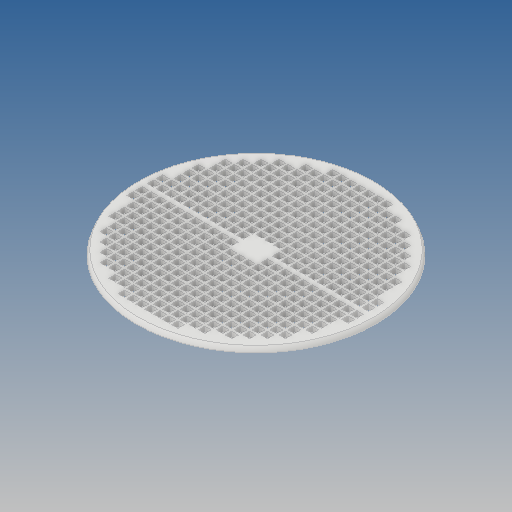
# Autodesk Inventor part: тело
Saved by Autodesk Inventor 2020 (Build 240168000, 168)
## iProperties
Created: 2019-09-06
Part Number: тело
Material: Пластик АБС
Document SubType Name: Modeling
Designer: Iliga
Density: 1.06 g/cm^3
Appearance: Гладкий — белый
Mass: 236.83 g
Surface Area: 2382.33 cm^2
Volume: 236.83 cm^3
Author: Iliga
Autodesk Inventor part; units mm, degrees
(part 1 of 3)
ref_plane "РабПлоскость1" through (0, -35, 0) normal (0, 1, 0) x (-1, 0, 0)
ref_plane "РабПлоскость7" through (100, -35, 0) normal (0, -1, 0) x (1, 0, 0)
ref_plane "YZ Plane" through (0, 0, 0) normal (1, 0, 0) x (0, 1, 0)
sketch "Эскиз118" plane through (0, 0, 0) normal (0, 0, 1) x (1, 0, 0)
  line L0 (0, 0) -> (-93.5, 0)
  line L1 (0, 4) -> (-91.9721, 4)
  line L2 (0, 4) -> (0, 0)
  line L3 (0, 45) -> (0, -57)
  arc A0 (-91.9721, 4) -> (-93.5, 0) centre (-87.5, 0) ccw
  point P0 (0, 2)
  dimension "d610" = 93.5
  dimension "d611" = 4
  dimension "d745" = 6
  constraints: 8 end point, 2 horizontal, 2 point on circle, 2 point on line, 2 vertical, 1 centre point, 1 midpoint
  measures "d610" distance of L0.start L0.end
  measures "d611" distance between parallel lines of L0 L1
  measures "d745" radius of A0
revolve "Вращение3" add sketch "Эскиз118" angle 270 about axis through (0, 45, 0) along (0, -1, 0)
sketch "Эскиз119" plane through (-91.9721, 4, 0) normal (0, 1, 0) x (1, 0, 0)
  line L0 (4.9721, 2) -> (9.9721, 2)
  line L1 (9.9721, 2) -> (9.9721, 7)
  line L2 (9.9721, 7) -> (4.9721, 7)
  line L3 (4.9721, 7) -> (4.9721, 2)
  line L4 (0, 0) -> (91.9721, 0) projected
  line L5 (91.9721, -91.9721) -> (91.9721, 0) projected
  line L6 (11.9721, 2) -> (16.9721, 2)
  line L7 (16.9721, 2) -> (16.9721, 7)
  line L8 (16.9721, 7) -> (11.9721, 7)
  line L9 (11.9721, 7) -> (11.9721, 2)
  line L10 (18.9721, 2) -> (23.9721, 2)
  line L11 (23.9721, 2) -> (23.9721, 7)
  line L12 (23.9721, 7) -> (18.9721, 7)
  line L13 (18.9721, 7) -> (18.9721, 2)
  line L14 (25.9721, 2) -> (30.9721, 2)
  line L15 (30.9721, 2) -> (30.9721, 7)
  line L16 (30.9721, 7) -> (25.9721, 7)
  line L17 (25.9721, 7) -> (25.9721, 2)
  line L18 (32.9721, 2) -> (37.9721, 2)
  line L19 (37.9721, 2) -> (37.9721, 7)
  line L20 (37.9721, 7) -> (32.9721, 7)
  line L21 (32.9721, 7) -> (32.9721, 2)
  line L22 (39.9721, 2) -> (44.9721, 2)
  line L23 (44.9721, 2) -> (44.9721, 7)
  line L24 (44.9721, 7) -> (39.9721, 7)
  line L25 (39.9721, 7) -> (39.9721, 2)
  line L26 (46.9721, 2) -> (51.9721, 2)
  line L27 (51.9721, 2) -> (51.9721, 7)
  line L28 (51.9721, 7) -> (46.9721, 7)
  line L29 (46.9721, 7) -> (46.9721, 2)
  line L30 (53.9721, 2) -> (58.9721, 2)
  line L31 (58.9721, 2) -> (58.9721, 7)
  line L32 (58.9721, 7) -> (53.9721, 7)
  line L33 (53.9721, 7) -> (53.9721, 2)
  line L34 (60.9721, 2) -> (65.9721, 2)
  line L35 (65.9721, 2) -> (65.9721, 7)
  line L36 (65.9721, 7) -> (60.9721, 7)
  line L37 (60.9721, 7) -> (60.9721, 2)
  line L38 (67.9721, 2) -> (72.9721, 2)
  line L39 (72.9721, 2) -> (72.9721, 7)
  line L40 (72.9721, 7) -> (67.9721, 7)
  line L41 (67.9721, 7) -> (67.9721, 2)
  line L42 (74.9721, 2) -> (79.9721, 2)
  line L43 (79.9721, 2) -> (79.9721, 7)
  line L44 (79.9721, 7) -> (74.9721, 7)
  line L45 (74.9721, 7) -> (74.9721, 2)
  line L46 (81.9721, 2) -> (86.9721, 2)
  line L47 (86.9721, 2) -> (86.9721, 7)
  line L48 (86.9721, 7) -> (81.9721, 7)
  line L49 (81.9721, 7) -> (81.9721, 2)
  line L50 (88.9721, 2) -> (93.9721, 2)
  line L51 (93.9721, 2) -> (93.9721, 7)
  line L52 (93.9721, 7) -> (88.9721, 7)
  line L53 (88.9721, 7) -> (88.9721, 2)
  line L54 (95.9721, 2) -> (100.9721, 2)
  line L55 (100.9721, 2) -> (100.9721, 7)
  line L56 (100.9721, 7) -> (95.9721, 7)
  line L57 (95.9721, 7) -> (95.9721, 2)
  line L58 (102.9721, 2) -> (107.9721, 2)
  line L59 (107.9721, 2) -> (107.9721, 7)
  line L60 (107.9721, 7) -> (102.9721, 7)
  line L61 (102.9721, 7) -> (102.9721, 2)
  line L62 (109.9721, 2) -> (114.9721, 2)
  line L63 (114.9721, 2) -> (114.9721, 7)
  line L64 (114.9721, 7) -> (109.9721, 7)
  line L65 (109.9721, 7) -> (109.9721, 2)
  line L66 (116.9721, 2) -> (121.9721, 2)
  line L67 (121.9721, 2) -> (121.9721, 7)
  line L68 (121.9721, 7) -> (116.9721, 7)
  line L69 (116.9721, 7) -> (116.9721, 2)
  line L70 (123.9721, 2) -> (128.9721, 2)
  line L71 (128.9721, 2) -> (128.9721, 7)
  line L72 (128.9721, 7) -> (123.9721, 7)
  line L73 (123.9721, 7) -> (123.9721, 2)
  line L74 (130.9721, 2) -> (135.9721, 2)
  line L75 (135.9721, 2) -> (135.9721, 7)
  line L76 (135.9721, 7) -> (130.9721, 7)
  line L77 (130.9721, 7) -> (130.9721, 2)
  line L78 (137.9721, 2) -> (142.9721, 2)
  line L79 (142.9721, 2) -> (142.9721, 7)
  line L80 (142.9721, 7) -> (137.9721, 7)
  line L81 (137.9721, 7) -> (137.9721, 2)
  line L82 (144.9721, 2) -> (149.9721, 2)
  line L83 (149.9721, 2) -> (149.9721, 7)
  line L84 (149.9721, 7) -> (144.9721, 7)
  line L85 (144.9721, 7) -> (144.9721, 2)
  line L86 (151.9721, 2) -> (156.9721, 2)
  line L87 (156.9721, 2) -> (156.9721, 7)
  line L88 (156.9721, 7) -> (151.9721, 7)
  line L89 (151.9721, 7) -> (151.9721, 2)
  line L90 (158.9721, 2) -> (163.9721, 2)
  line L91 (163.9721, 2) -> (163.9721, 7)
  line L92 (163.9721, 7) -> (158.9721, 7)
  line L93 (158.9721, 7) -> (158.9721, 2)
  line L94 (165.9721, 2) -> (170.9721, 2)
  line L95 (170.9721, 2) -> (170.9721, 7)
  line L96 (170.9721, 7) -> (165.9721, 7)
  line L97 (165.9721, 7) -> (165.9721, 2)
  line L98 (172.9721, 2) -> (177.9721, 2)
  line L99 (177.9721, 2) -> (177.9721, 7)
  line L100 (177.9721, 7) -> (172.9721, 7)
  line L101 (172.9721, 7) -> (172.9721, 2)
  line L102 (4.9721, 9) -> (9.9721, 9)
  line L103 (9.9721, 9) -> (9.9721, 14)
  line L104 (9.9721, 14) -> (4.9721, 14)
  line L105 (4.9721, 14) -> (4.9721, 9)
  line L106 (172.9721, 14) -> (172.9721, 9)
  line L107 (177.9721, 9) -> (177.9721, 14)
  line L108 (177.9721, 14) -> (172.9721, 14)
  line L109 (172.9721, 9) -> (177.9721, 9)
  line L110 (39.9721, 14) -> (39.9721, 9)
  line L111 (51.9721, 9) -> (51.9721, 14)
  line L112 (53.9721, 14) -> (53.9721, 9)
  line L113 (58.9721, 9) -> (58.9721, 14)
  line L114 (58.9721, 14) -> (53.9721, 14)
  line L115 (60.9721, 14) -> (60.9721, 9)
  line L116 (65.9721, 9) -> (65.9721, 14)
  line L117 (65.9721, 14) -> (60.9721, 14)
  line L118 (60.9721, 9) -> (65.9721, 9)
  line L119 (53.9721, 9) -> (58.9721, 9)
  line L120 (67.9721, 14) -> (67.9721, 9)
  line L121 (72.9721, 9) -> (72.9721, 14)
  line L122 (67.9721, 9) -> (72.9721, 9)
  line L123 (72.9721, 14) -> (67.9721, 14)
  line L124 (74.9721, 14) -> (74.9721, 9)
  line L125 (79.9721, 9) -> (79.9721, 14)
  line L126 (74.9721, 9) -> (79.9721, 9)
  line L127 (79.9721, 14) -> (74.9721, 14)
  line L128 (81.9721, 14) -> (81.9721, 9)
  line L129 (81.9721, 9) -> (86.9721, 9)
  line L130 (86.9721, 14) -> (81.9721, 14)
  line L131 (86.9721, 9) -> (86.9721, 14)
  line L132 (88.9721, 14) -> (88.9721, 9)
  line L133 (93.9721, 9) -> (93.9721, 14)
  line L134 (93.9721, 14) -> (88.9721, 14)
  line L135 (88.9721, 9) -> (93.9721, 9)
  line L136 (95.9721, 14) -> (95.9721, 9)
  line L137 (95.9721, 9) -> (100.9721, 9)
  line L138 (100.9721, 14) -> (95.9721, 14)
  line L139 (100.9721, 9) -> (100.9721, 14)
  line L140 (102.9721, 14) -> (102.9721, 9)
  line L141 (102.9721, 9) -> (107.9721, 9)
  line L142 (107.9721, 14) -> (102.9721, 14)
  line L143 (107.9721, 9) -> (107.9721, 14)
  line L144 (109.9721, 14) -> (109.9721, 9)
  line L145 (109.9721, 9) -> (114.9721, 9)
  line L146 (114.9721, 14) -> (109.9721, 14)
  line L147 (114.9721, 9) -> (114.9721, 14)
  line L148 (116.9721, 14) -> (116.9721, 9)
  line L149 (116.9721, 9) -> (121.9721, 9)
  line L150 (121.9721, 14) -> (116.9721, 14)
  line L151 (121.9721, 9) -> (121.9721, 14)
  line L152 (123.9721, 14) -> (123.9721, 9)
  line L153 (128.9721, 9) -> (128.9721, 14)
  line L154 (123.9721, 9) -> (128.9721, 9)
  line L155 (128.9721, 14) -> (123.9721, 14)
  line L156 (130.9721, 14) -> (130.9721, 9)
  line L157 (130.9721, 9) -> (135.9721, 9)
  line L158 (135.9721, 14) -> (130.9721, 14)
  line L159 (135.9721, 9) -> (135.9721, 14)
  line L160 (137.9721, 14) -> (137.9721, 9)
  line L161 (137.9721, 9) -> (142.9721, 9)
  line L162 (142.9721, 14) -> (137.9721, 14)
  line L163 (142.9721, 9) -> (142.9721, 14)
  line L164 (144.9721, 14) -> (144.9721, 9)
  line L165 (144.9721, 9) -> (149.9721, 9)
  line L166 (149.9721, 14) -> (144.9721, 14)
  line L167 (149.9721, 9) -> (149.9721, 14)
  line L168 (151.9721, 14) -> (151.9721, 9)
  line L169 (151.9721, 9) -> (156.9721, 9)
  line L170 (156.9721, 14) -> (151.9721, 14)
  line L171 (158.9721, 14) -> (158.9721, 9)
  line L172 (163.9721, 9) -> (163.9721, 14)
  line L173 (163.9721, 14) -> (158.9721, 14)
  line L174 (158.9721, 9) -> (163.9721, 9)
  line L175 (156.9721, 9) -> (156.9721, 14)
  line L176 (165.9721, 14) -> (165.9721, 9)
  line L177 (170.9721, 14) -> (165.9721, 14)
  line L178 (165.9721, 9) -> (170.9721, 9)
  line L179 (170.9721, 9) -> (170.9721, 14)
  line L180 (11.9721, 14) -> (11.9721, 9)
  line L181 (16.9721, 14) -> (11.9721, 14)
  line L182 (16.9721, 9) -> (16.9721, 14)
  line L183 (18.9721, 14) -> (18.9721, 9)
  line L184 (23.9721, 14) -> (18.9721, 14)
  line L185 (23.9721, 9) -> (23.9721, 14)
  line L186 (18.9721, 9) -> (23.9721, 9)
  line L187 (11.9721, 9) -> (16.9721, 9)
  line L188 (37.9721, 9) -> (37.9721, 14)
  line L189 (44.9721, 9) -> (44.9721, 14)
  line L190 (39.9721, 9) -> (44.9721, 9)
  line L191 (44.9721, 14) -> (39.9721, 14)
  line L192 (46.9721, 14) -> (46.9721, 9)
  line L193 (32.9721, 9) -> (37.9721, 9)
  line L194 (37.9721, 14) -> (32.9721, 14)
  line L195 (32.9721, 14) -> (32.9721, 9)
  line L196 (30.9721, 9) -> (30.9721, 14)
  line L197 (46.9721, 9) -> (51.9721, 9)
  line L198 (51.9721, 14) -> (46.9721, 14)
  line L199 (25.9721, 9) -> (30.9721, 9)
  line L200 (30.9721, 14) -> (25.9721, 14)
  line L201 (25.9721, 14) -> (25.9721, 9)
  line L202 (39.9721, 21) -> (39.9721, 16)
  line L203 (51.9721, 16) -> (51.9721, 21)
  line L204 (53.9721, 21) -> (53.9721, 16)
  line L205 (58.9721, 16) -> (58.9721, 21)
  line L206 (58.9721, 21) -> (53.9721, 21)
  line L207 (60.9721, 21) -> (60.9721, 16)
  line L208 (65.9721, 16) -> (65.9721, 21)
  line L209 (65.9721, 21) -> (60.9721, 21)
  line L210 (60.9721, 16) -> (65.9721, 16)
  line L211 (53.9721, 16) -> (58.9721, 16)
  line L212 (67.9721, 21) -> (67.9721, 16)
  line L213 (72.9721, 16) -> (72.9721, 21)
  line L214 (67.9721, 16) -> (72.9721, 16)
  line L215 (72.9721, 21) -> (67.9721, 21)
  line L216 (74.9721, 21) -> (74.9721, 16)
  line L217 (79.9721, 16) -> (79.9721, 21)
  line L218 (74.9721, 16) -> (79.9721, 16)
  line L219 (79.9721, 21) -> (74.9721, 21)
  line L220 (81.9721, 21) -> (81.9721, 16)
  line L221 (81.9721, 16) -> (86.9721, 16)
  line L222 (86.9721, 21) -> (81.9721, 21)
  line L223 (86.9721, 16) -> (86.9721, 21)
  line L224 (88.9721, 21) -> (88.9721, 16)
  line L225 (93.9721, 16) -> (93.9721, 21)
  line L226 (93.9721, 21) -> (88.9721, 21)
  line L227 (88.9721, 16) -> (93.9721, 16)
  line L228 (95.9721, 21) -> (95.9721, 16)
  line L229 (95.9721, 16) -> (100.9721, 16)
  line L230 (100.9721, 21) -> (95.9721, 21)
  line L231 (100.9721, 16) -> (100.9721, 21)
  line L232 (102.9721, 21) -> (102.9721, 16)
  line L233 (102.9721, 16) -> (107.9721, 16)
  line L234 (107.9721, 21) -> (102.9721, 21)
  line L235 (107.9721, 16) -> (107.9721, 21)
  line L236 (109.9721, 21) -> (109.9721, 16)
  line L237 (109.9721, 16) -> (114.9721, 16)
  line L238 (114.9721, 21) -> (109.9721, 21)
  line L239 (114.9721, 16) -> (114.9721, 21)
  line L240 (116.9721, 21) -> (116.9721, 16)
  line L241 (116.9721, 16) -> (121.9721, 16)
  line L242 (121.9721, 21) -> (116.9721, 21)
  line L243 (121.9721, 16) -> (121.9721, 21)
  line L244 (123.9721, 21) -> (123.9721, 16)
  line L245 (128.9721, 16) -> (128.9721, 21)
  line L246 (123.9721, 16) -> (128.9721, 16)
  line L247 (128.9721, 21) -> (123.9721, 21)
  line L248 (130.9721, 21) -> (130.9721, 16)
  line L249 (130.9721, 16) -> (135.9721, 16)
  line L250 (135.9721, 21) -> (130.9721, 21)
  line L251 (135.9721, 16) -> (135.9721, 21)
  line L252 (137.9721, 21) -> (137.9721, 16)
  line L253 (137.9721, 16) -> (142.9721, 16)
  line L254 (142.9721, 21) -> (137.9721, 21)
  line L255 (142.9721, 16) -> (142.9721, 21)
  line L256 (144.9721, 21) -> (144.9721, 16)
  line L257 (144.9721, 16) -> (149.9721, 16)
  line L258 (149.9721, 21) -> (144.9721, 21)
  line L259 (149.9721, 16) -> (149.9721, 21)
  line L260 (151.9721, 21) -> (151.9721, 16)
  line L261 (151.9721, 16) -> (156.9721, 16)
  line L262 (156.9721, 21) -> (151.9721, 21)
  line L263 (158.9721, 21) -> (158.9721, 16)
  line L264 (163.9721, 16) -> (163.9721, 21)
  line L265 (163.9721, 21) -> (158.9721, 21)
  line L266 (158.9721, 16) -> (163.9721, 16)
  line L267 (156.9721, 16) -> (156.9721, 21)
  line L268 (165.9721, 21) -> (165.9721, 16)
  line L269 (170.9721, 21) -> (165.9721, 21)
  line L270 (165.9721, 16) -> (170.9721, 16)
  line L271 (170.9721, 16) -> (170.9721, 21)
  line L272 (11.9721, 21) -> (11.9721, 16)
  line L273 (16.9721, 21) -> (11.9721, 21)
  line L274 (16.9721, 16) -> (16.9721, 21)
  line L275 (18.9721, 21) -> (18.9721, 16)
  line L276 (23.9721, 21) -> (18.9721, 21)
  line L277 (23.9721, 16) -> (23.9721, 21)
  line L278 (18.9721, 16) -> (23.9721, 16)
  line L279 (11.9721, 16) -> (16.9721, 16)
  line L280 (37.9721, 16) -> (37.9721, 21)
  line L281 (44.9721, 16) -> (44.9721, 21)
  line L282 (39.9721, 16) -> (44.9721, 16)
  line L283 (44.9721, 21) -> (39.9721, 21)
  line L284 (46.9721, 21) -> (46.9721, 16)
  line L285 (32.9721, 16) -> (37.9721, 16)
  line L286 (37.9721, 21) -> (32.9721, 21)
  line L287 (32.9721, 21) -> (32.9721, 16)
  line L288 (30.9721, 16) -> (30.9721, 21)
  line L289 (46.9721, 16) -> (51.9721, 16)
  line L290 (51.9721, 21) -> (46.9721, 21)
  line L291 (25.9721, 16) -> (30.9721, 16)
  line L292 (30.9721, 21) -> (25.9721, 21)
  line L293 (25.9721, 21) -> (25.9721, 16)
  line L294 (39.9721, 28) -> (39.9721, 23)
  line L295 (51.9721, 23) -> (51.9721, 28)
  line L296 (53.9721, 28) -> (53.9721, 23)
  line L297 (58.9721, 23) -> (58.9721, 28)
  line L298 (58.9721, 28) -> (53.9721, 28)
  line L299 (60.9721, 28) -> (60.9721, 23)
  line L300 (65.9721, 23) -> (65.9721, 28)
  line L301 (65.9721, 28) -> (60.9721, 28)
  line L302 (60.9721, 23) -> (65.9721, 23)
  line L303 (53.9721, 23) -> (58.9721, 23)
  line L304 (67.9721, 28) -> (67.9721, 23)
  line L305 (72.9721, 23) -> (72.9721, 28)
  line L306 (67.9721, 23) -> (72.9721, 23)
  line L307 (72.9721, 28) -> (67.9721, 28)
  line L308 (74.9721, 28) -> (74.9721, 23)
  line L309 (79.9721, 23) -> (79.9721, 28)
  line L310 (74.9721, 23) -> (79.9721, 23)
  line L311 (79.9721, 28) -> (74.9721, 28)
  line L312 (81.9721, 28) -> (81.9721, 23)
  line L313 (81.9721, 23) -> (86.9721, 23)
  line L314 (86.9721, 28) -> (81.9721, 28)
  line L315 (86.9721, 23) -> (86.9721, 28)
  line L316 (88.9721, 28) -> (88.9721, 23)
  line L317 (93.9721, 23) -> (93.9721, 28)
  line L318 (93.9721, 28) -> (88.9721, 28)
  line L319 (88.9721, 23) -> (93.9721, 23)
  line L320 (95.9721, 28) -> (95.9721, 23)
  line L321 (95.9721, 23) -> (100.9721, 23)
  line L322 (100.9721, 28) -> (95.9721, 28)
  line L323 (100.9721, 23) -> (100.9721, 28)
  line L324 (102.9721, 28) -> (102.9721, 23)
  line L325 (102.9721, 23) -> (107.9721, 23)
  line L326 (107.9721, 28) -> (102.9721, 28)
  line L327 (107.9721, 23) -> (107.9721, 28)
  line L328 (109.9721, 28) -> (109.9721, 23)
  line L329 (109.9721, 23) -> (114.9721, 23)
  line L330 (114.9721, 28) -> (109.9721, 28)
  line L331 (114.9721, 23) -> (114.9721, 28)
  line L332 (116.9721, 28) -> (116.9721, 23)
  line L333 (116.9721, 23) -> (121.9721, 23)
  line L334 (121.9721, 28) -> (116.9721, 28)
  line L335 (121.9721, 23) -> (121.9721, 28)
  line L336 (123.9721, 28) -> (123.9721, 23)
  line L337 (128.9721, 23) -> (128.9721, 28)
  line L338 (123.9721, 23) -> (128.9721, 23)
  line L339 (128.9721, 28) -> (123.9721, 28)
  line L340 (130.9721, 28) -> (130.9721, 23)
  line L341 (130.9721, 23) -> (135.9721, 23)
  line L342 (135.9721, 28) -> (130.9721, 28)
  line L343 (135.9721, 23) -> (135.9721, 28)
  line L344 (137.9721, 28) -> (137.9721, 23)
  line L345 (137.9721, 23) -> (142.9721, 23)
  line L346 (142.9721, 28) -> (137.9721, 28)
  line L347 (142.9721, 23) -> (142.9721, 28)
  line L348 (144.9721, 28) -> (144.9721, 23)
  line L349 (144.9721, 23) -> (149.9721, 23)
  line L350 (149.9721, 28) -> (144.9721, 28)
  line L351 (149.9721, 23) -> (149.9721, 28)
  line L352 (151.9721, 28) -> (151.9721, 23)
  line L353 (151.9721, 23) -> (156.9721, 23)
  line L354 (156.9721, 28) -> (151.9721, 28)
  line L355 (158.9721, 28) -> (158.9721, 23)
  line L356 (163.9721, 23) -> (163.9721, 28)
  line L357 (163.9721, 28) -> (158.9721, 28)
  line L358 (158.9721, 23) -> (163.9721, 23)
  line L359 (156.9721, 23) -> (156.9721, 28)
  line L360 (165.9721, 28) -> (165.9721, 23)
  line L361 (170.9721, 28) -> (165.9721, 28)
  line L362 (165.9721, 23) -> (170.9721, 23)
  line L363 (170.9721, 23) -> (170.9721, 28)
  line L364 (11.9721, 28) -> (11.9721, 23)
  line L365 (16.9721, 28) -> (11.9721, 28)
  line L366 (16.9721, 23) -> (16.9721, 28)
  line L367 (18.9721, 28) -> (18.9721, 23)
  line L368 (23.9721, 28) -> (18.9721, 28)
  line L369 (23.9721, 23) -> (23.9721, 28)
  line L370 (18.9721, 23) -> (23.9721, 23)
  line L371 (11.9721, 23) -> (16.9721, 23)
  line L372 (37.9721, 23) -> (37.9721, 28)
  line L373 (44.9721, 23) -> (44.9721, 28)
  line L374 (39.9721, 23) -> (44.9721, 23)
  line L375 (44.9721, 28) -> (39.9721, 28)
  line L376 (46.9721, 28) -> (46.9721, 23)
  line L377 (32.9721, 23) -> (37.9721, 23)
  line L378 (37.9721, 28) -> (32.9721, 28)
  line L379 (32.9721, 28) -> (32.9721, 23)
  line L380 (30.9721, 23) -> (30.9721, 28)
  line L381 (46.9721, 23) -> (51.9721, 23)
  line L382 (51.9721, 28) -> (46.9721, 28)
  line L383 (25.9721, 23) -> (30.9721, 23)
  line L384 (30.9721, 28) -> (25.9721, 28)
  line L385 (25.9721, 28) -> (25.9721, 23)
  line L386 (39.9721, 35) -> (39.9721, 30)
  line L387 (51.9721, 30) -> (51.9721, 35)
  line L388 (53.9721, 35) -> (53.9721, 30)
  line L389 (58.9721, 30) -> (58.9721, 35)
  line L390 (58.9721, 35) -> (53.9721, 35)
  line L391 (60.9721, 35) -> (60.9721, 30)
  line L392 (65.9721, 30) -> (65.9721, 35)
  line L393 (65.9721, 35) -> (60.9721, 35)
  line L394 (60.9721, 30) -> (65.9721, 30)
  line L395 (53.9721, 30) -> (58.9721, 30)
  line L396 (67.9721, 35) -> (67.9721, 30)
  line L397 (72.9721, 30) -> (72.9721, 35)
  line L398 (67.9721, 30) -> (72.9721, 30)
  line L399 (72.9721, 35) -> (67.9721, 35)
  line L400 (74.9721, 35) -> (74.9721, 30)
  line L401 (79.9721, 30) -> (79.9721, 35)
  line L402 (74.9721, 30) -> (79.9721, 30)
  line L403 (79.9721, 35) -> (74.9721, 35)
  line L404 (81.9721, 35) -> (81.9721, 30)
  line L405 (81.9721, 30) -> (86.9721, 30)
  line L406 (86.9721, 35) -> (81.9721, 35)
  line L407 (86.9721, 30) -> (86.9721, 35)
  line L408 (88.9721, 35) -> (88.9721, 30)
  line L409 (93.9721, 30) -> (93.9721, 35)
  line L410 (93.9721, 35) -> (88.9721, 35)
  line L411 (88.9721, 30) -> (93.9721, 30)
  line L412 (95.9721, 35) -> (95.9721, 30)
  line L413 (95.9721, 30) -> (100.9721, 30)
  line L414 (100.9721, 35) -> (95.9721, 35)
  line L415 (100.9721, 30) -> (100.9721, 35)
  line L416 (102.9721, 35) -> (102.9721, 30)
  line L417 (102.9721, 30) -> (107.9721, 30)
  line L418 (107.9721, 35) -> (102.9721, 35)
  line L419 (107.9721, 30) -> (107.9721, 35)
  line L420 (109.9721, 35) -> (109.9721, 30)
  line L421 (109.9721, 30) -> (114.9721, 30)
  line L422 (114.9721, 35) -> (109.9721, 35)
  line L423 (114.9721, 30) -> (114.9721, 35)
  line L424 (116.9721, 35) -> (116.9721, 30)
  line L425 (116.9721, 30) -> (121.9721, 30)
  line L426 (121.9721, 35) -> (116.9721, 35)
  line L427 (121.9721, 30) -> (121.9721, 35)
  line L428 (123.9721, 35) -> (123.9721, 30)
  line L429 (128.9721, 30) -> (128.9721, 35)
  line L430 (123.9721, 30) -> (128.9721, 30)
  line L431 (128.9721, 35) -> (123.9721, 35)
  line L432 (130.9721, 35) -> (130.9721, 30)
  line L433 (130.9721, 30) -> (135.9721, 30)
  line L434 (135.9721, 35) -> (130.9721, 35)
  line L435 (135.9721, 30) -> (135.9721, 35)
  line L436 (137.9721, 35) -> (137.9721, 30)
  line L437 (137.9721, 30) -> (142.9721, 30)
  line L438 (142.9721, 35) -> (137.9721, 35)
  line L439 (142.9721, 30) -> (142.9721, 35)
  line L440 (144.9721, 35) -> (144.9721, 30)
  line L441 (144.9721, 30) -> (149.9721, 30)
  line L442 (149.9721, 35) -> (144.9721, 35)
  line L443 (149.9721, 30) -> (149.9721, 35)
  line L444 (151.9721, 35) -> (151.9721, 30)
  line L445 (151.9721, 30) -> (156.9721, 30)
  line L446 (156.9721, 35) -> (151.9721, 35)
  line L447 (158.9721, 35) -> (158.9721, 30)
  line L448 (163.9721, 30) -> (163.9721, 35)
  line L449 (163.9721, 35) -> (158.9721, 35)
  line L450 (158.9721, 30) -> (163.9721, 30)
  line L451 (156.9721, 30) -> (156.9721, 35)
  line L452 (165.9721, 35) -> (165.9721, 30)
  line L453 (170.9721, 35) -> (165.9721, 35)
  line L454 (165.9721, 30) -> (170.9721, 30)
  line L455 (170.9721, 30) -> (170.9721, 35)
  line L456 (11.9721, 35) -> (11.9721, 30)
  line L457 (16.9721, 35) -> (11.9721, 35)
  line L458 (16.9721, 30) -> (16.9721, 35)
  line L459 (18.9721, 35) -> (18.9721, 30)
  line L460 (23.9721, 35) -> (18.9721, 35)
  line L461 (23.9721, 30) -> (23.9721, 35)
  line L462 (18.9721, 30) -> (23.9721, 30)
  line L463 (11.9721, 30) -> (16.9721, 30)
  line L464 (37.9721, 30) -> (37.9721, 35)
  line L465 (44.9721, 30) -> (44.9721, 35)
  line L466 (39.9721, 30) -> (44.9721, 30)
  line L467 (44.9721, 35) -> (39.9721, 35)
  line L468 (46.9721, 35) -> (46.9721, 30)
  line L469 (32.9721, 30) -> (37.9721, 30)
  line L470 (37.9721, 35) -> (32.9721, 35)
  line L471 (32.9721, 35) -> (32.9721, 30)
  line L472 (30.9721, 30) -> (30.9721, 35)
  line L473 (46.9721, 30) -> (51.9721, 30)
  line L474 (51.9721, 35) -> (46.9721, 35)
  line L475 (25.9721, 30) -> (30.9721, 30)
  line L476 (30.9721, 35) -> (25.9721, 35)
  line L477 (25.9721, 35) -> (25.9721, 30)
  line L478 (72.9721, 42) -> (67.9721, 42)
  line L479 (67.9721, 42) -> (67.9721, 37)
  line L480 (72.9721, 37) -> (72.9721, 42)
  line L481 (74.9721, 42) -> (74.9721, 37)
  line L482 (74.9721, 37) -> (79.9721, 37)
  line L483 (79.9721, 42) -> (74.9721, 42)
  line L484 (79.9721, 37) -> (79.9721, 42)
  line L485 (53.9721, 42) -> (53.9721, 37)
  line L486 (58.9721, 42) -> (53.9721, 42)
  line L487 (53.9721, 37) -> (58.9721, 37)
  line L488 (58.9721, 37) -> (58.9721, 42)
  line L489 (60.9721, 42) -> (60.9721, 37)
  line L490 (65.9721, 37) -> (65.9721, 42)
  line L491 (65.9721, 42) -> (60.9721, 42)
  line L492 (60.9721, 37) -> (65.9721, 37)
  line L493 (46.9721, 37) -> (51.9721, 37)
  line L494 (44.9721, 37) -> (44.9721, 42)
  line L495 (46.9721, 42) -> (46.9721, 37)
  line L496 (51.9721, 42) -> (46.9721, 42)
  line L497 (51.9721, 37) -> (51.9721, 42)
  line L498 (25.9721, 42) -> (25.9721, 37)
  line L499 (30.9721, 37) -> (30.9721, 42)
  line L500 (30.9721, 42) -> (25.9721, 42)
  line L501 (25.9721, 37) -> (30.9721, 37)
  line L502 (18.9721, 37) -> (23.9721, 37)
  line L503 (23.9721, 37) -> (23.9721, 42)
  line L504 (18.9721, 42) -> (18.9721, 37)
  line L505 (23.9721, 42) -> (18.9721, 42)
  line L506 (39.9721, 37) -> (44.9721, 37)
  line L507 (44.9721, 42) -> (39.9721, 42)
  line L508 (39.9721, 42) -> (39.9721, 37)
  line L509 (37.9721, 37) -> (37.9721, 42)
  line L510 (32.9721, 42) -> (32.9721, 37)
  line L511 (37.9721, 42) -> (32.9721, 42)
  line L512 (32.9721, 37) -> (37.9721, 37)
  line L513 (88.9721, 37) -> (93.9721, 37)
  line L514 (81.9721, 37) -> (86.9721, 37)
  line L515 (93.9721, 37) -> (93.9721, 42)
  line L516 (93.9721, 42) -> (88.9721, 42)
  line L517 (88.9721, 42) -> (88.9721, 37)
  line L518 (86.9721, 37) -> (86.9721, 42)
  line L519 (86.9721, 42) -> (81.9721, 42)
  line L520 (81.9721, 42) -> (81.9721, 37)
  line L521 (102.9721, 37) -> (107.9721, 37)
  line L522 (109.9721, 42) -> (109.9721, 37)
  line L523 (107.9721, 42) -> (102.9721, 42)
  line L524 (107.9721, 37) -> (107.9721, 42)
  line L525 (102.9721, 42) -> (102.9721, 37)
  line L526 (100.9721, 37) -> (100.9721, 42)
  line L527 (95.9721, 42) -> (95.9721, 37)
  line L528 (100.9721, 42) -> (95.9721, 42)
  line L529 (95.9721, 37) -> (100.9721, 37)
  line L530 (116.9721, 37) -> (121.9721, 37)
  line L531 (116.9721, 42) -> (116.9721, 37)
  line L532 (121.9721, 42) -> (116.9721, 42)
  line L533 (114.9721, 37) -> (114.9721, 42)
  line L534 (109.9721, 37) -> (114.9721, 37)
  line L535 (114.9721, 42) -> (109.9721, 42)
  line L536 (123.9721, 37) -> (128.9721, 37)
  line L537 (121.9721, 37) -> (121.9721, 42)
  line L538 (123.9721, 42) -> (123.9721, 37)
  line L539 (128.9721, 42) -> (123.9721, 42)
  line L540 (67.9721, 37) -> (72.9721, 37)
  line L541 (130.9721, 37) -> (135.9721, 37)
  line L542 (137.9721, 37) -> (142.9721, 37)
  line L543 (130.9721, 42) -> (130.9721, 37)
  line L544 (135.9721, 42) -> (130.9721, 42)
  line L545 (128.9721, 37) -> (128.9721, 42)
  line L546 (135.9721, 37) -> (135.9721, 42)
  line L547 (137.9721, 42) -> (137.9721, 37)
  line L548 (142.9721, 42) -> (137.9721, 42)
  line L549 (151.9721, 42) -> (151.9721, 37)
  line L550 (151.9721, 37) -> (156.9721, 37)
  line L551 (156.9721, 37) -> (156.9721, 42)
  line L552 (156.9721, 42) -> (151.9721, 42)
  line L553 (158.9721, 37) -> (163.9721, 37)
  line L554 (163.9721, 37) -> (163.9721, 42)
  line L555 (158.9721, 42) -> (158.9721, 37)
  line L556 (163.9721, 42) -> (158.9721, 42)
  line L557 (149.9721, 37) -> (149.9721, 42)
  line L558 (144.9721, 42) -> (144.9721, 37)
  line L559 (149.9721, 42) -> (144.9721, 42)
  line L560 (142.9721, 37) -> (142.9721, 42)
  line L561 (144.9721, 37) -> (149.9721, 37)
  line L562 (72.9721, 49) -> (67.9721, 49)
  line L563 (67.9721, 49) -> (67.9721, 44)
  line L564 (72.9721, 44) -> (72.9721, 49)
  line L565 (74.9721, 49) -> (74.9721, 44)
  line L566 (74.9721, 44) -> (79.9721, 44)
  line L567 (79.9721, 49) -> (74.9721, 49)
  line L568 (79.9721, 44) -> (79.9721, 49)
  line L569 (53.9721, 49) -> (53.9721, 44)
  line L570 (58.9721, 49) -> (53.9721, 49)
  line L571 (53.9721, 44) -> (58.9721, 44)
  line L572 (58.9721, 44) -> (58.9721, 49)
  line L573 (60.9721, 49) -> (60.9721, 44)
  line L574 (65.9721, 44) -> (65.9721, 49)
  line L575 (65.9721, 49) -> (60.9721, 49)
  line L576 (60.9721, 44) -> (65.9721, 44)
  line L577 (46.9721, 44) -> (51.9721, 44)
  line L578 (44.9721, 44) -> (44.9721, 49)
  line L579 (46.9721, 49) -> (46.9721, 44)
  line L580 (51.9721, 49) -> (46.9721, 49)
  line L581 (51.9721, 44) -> (51.9721, 49)
  line L582 (25.9721, 49) -> (25.9721, 44)
  line L583 (30.9721, 44) -> (30.9721, 49)
  line L584 (30.9721, 49) -> (25.9721, 49)
  line L585 (25.9721, 44) -> (30.9721, 44)
  line L586 (18.9721, 44) -> (23.9721, 44)
  line L587 (23.9721, 44) -> (23.9721, 49)
  line L588 (18.9721, 49) -> (18.9721, 44)
  line L589 (23.9721, 49) -> (18.9721, 49)
  line L590 (39.9721, 44) -> (44.9721, 44)
  line L591 (44.9721, 49) -> (39.9721, 49)
  line L592 (39.9721, 49) -> (39.9721, 44)
  line L593 (37.9721, 44) -> (37.9721, 49)
  line L594 (32.9721, 49) -> (32.9721, 44)
  line L595 (37.9721, 49) -> (32.9721, 49)
  line L596 (32.9721, 44) -> (37.9721, 44)
  line L597 (88.9721, 44) -> (93.9721, 44)
  line L598 (81.9721, 44) -> (86.9721, 44)
  line L599 (93.9721, 44) -> (93.9721, 49)
  line L600 (93.9721, 49) -> (88.9721, 49)
  line L601 (88.9721, 49) -> (88.9721, 44)
  line L602 (86.9721, 44) -> (86.9721, 49)
  line L603 (86.9721, 49) -> (81.9721, 49)
  line L604 (81.9721, 49) -> (81.9721, 44)
  line L605 (102.9721, 44) -> (107.9721, 44)
  line L606 (109.9721, 49) -> (109.9721, 44)
  line L607 (107.9721, 49) -> (102.9721, 49)
  line L608 (107.9721, 44) -> (107.9721, 49)
  line L609 (102.9721, 49) -> (102.9721, 44)
  line L610 (100.9721, 44) -> (100.9721, 49)
  line L611 (95.9721, 49) -> (95.9721, 44)
  line L612 (100.9721, 49) -> (95.9721, 49)
  line L613 (95.9721, 44) -> (100.9721, 44)
  line L614 (116.9721, 44) -> (121.9721, 44)
  line L615 (116.9721, 49) -> (116.9721, 44)
  line L616 (121.9721, 49) -> (116.9721, 49)
  line L617 (114.9721, 44) -> (114.9721, 49)
  line L618 (109.9721, 44) -> (114.9721, 44)
  line L619 (114.9721, 49) -> (109.9721, 49)
  line L620 (123.9721, 44) -> (128.9721, 44)
  line L621 (121.9721, 44) -> (121.9721, 49)
  line L622 (123.9721, 49) -> (123.9721, 44)
  line L623 (128.9721, 49) -> (123.9721, 49)
  line L624 (67.9721, 44) -> (72.9721, 44)
  line L625 (130.9721, 44) -> (135.9721, 44)
  line L626 (137.9721, 44) -> (142.9721, 44)
  line L627 (130.9721, 49) -> (130.9721, 44)
  line L628 (135.9721, 49) -> (130.9721, 49)
  line L629 (128.9721, 44) -> (128.9721, 49)
  line L630 (135.9721, 44) -> (135.9721, 49)
  line L631 (137.9721, 49) -> (137.9721, 44)
  line L632 (142.9721, 49) -> (137.9721, 49)
  line L633 (151.9721, 49) -> (151.9721, 44)
  line L634 (151.9721, 44) -> (156.9721, 44)
  line L635 (156.9721, 44) -> (156.9721, 49)
  line L636 (156.9721, 49) -> (151.9721, 49)
  line L637 (158.9721, 44) -> (163.9721, 44)
  line L638 (163.9721, 44) -> (163.9721, 49)
  line L639 (158.9721, 49) -> (158.9721, 44)
  line L640 (163.9721, 49) -> (158.9721, 49)
  line L641 (149.9721, 44) -> (149.9721, 49)
  line L642 (144.9721, 49) -> (144.9721, 44)
  line L643 (149.9721, 49) -> (144.9721, 49)
  line L644 (142.9721, 44) -> (142.9721, 49)
  line L645 (144.9721, 44) -> (149.9721, 44)
  line L646 (65.9721, 51) -> (65.9721, 56)
  line L647 (60.9721, 51) -> (65.9721, 51)
  line L648 (65.9721, 56) -> (60.9721, 56)
  line L649 (60.9721, 56) -> (60.9721, 51)
  line L650 (58.9721, 51) -> (58.9721, 56)
  line L651 (46.9721, 51) -> (51.9721, 51)
  line L652 (51.9721, 56) -> (46.9721, 56)
  line L653 (39.9721, 51) -> (44.9721, 51)
  line L654 (46.9721, 56) -> (46.9721, 51)
  line L655 (44.9721, 51) -> (44.9721, 56)
  line L656 (39.9721, 56) -> (39.9721, 51)
  line L657 (44.9721, 56) -> (39.9721, 56)
  line L658 (37.9721, 51) -> (37.9721, 56)
  line L659 (37.9721, 56) -> (32.9721, 56)
  line L660 (32.9721, 51) -> (37.9721, 51)
  line L661 (25.9721, 51) -> (30.9721, 51)
  line L662 (25.9721, 56) -> (25.9721, 51)
  line L663 (30.9721, 56) -> (25.9721, 56)
  line L664 (30.9721, 51) -> (30.9721, 56)
  line L665 (32.9721, 56) -> (32.9721, 51)
  line L666 (53.9721, 56) -> (53.9721, 51)
  line L667 (53.9721, 51) -> (58.9721, 51)
  line L668 (58.9721, 56) -> (53.9721, 56)
  line L669 (51.9721, 51) -> (51.9721, 56)
  line L670 (149.9721, 51) -> (149.9721, 56)
  line L671 (144.9721, 51) -> (149.9721, 51)
  line L672 (149.9721, 56) -> (144.9721, 56)
  line L673 (151.9721, 56) -> (151.9721, 51)
  line L674 (142.9721, 56) -> (137.9721, 56)
  line L675 (142.9721, 51) -> (142.9721, 56)
  line L676 (144.9721, 56) -> (144.9721, 51)
  line L677 (137.9721, 51) -> (142.9721, 51)
  line L678 (137.9721, 56) -> (137.9721, 51)
  line L679 (130.9721, 51) -> (135.9721, 51)
  line L680 (135.9721, 51) -> (135.9721, 56)
  line L681 (130.9721, 56) -> (130.9721, 51)
  line L682 (135.9721, 56) -> (130.9721, 56)
  line L683 (116.9721, 51) -> (121.9721, 51)
  line L684 (116.9721, 56) -> (116.9721, 51)
  line L685 (121.9721, 56) -> (116.9721, 56)
  line L686 (121.9721, 51) -> (121.9721, 56)
  line L687 (123.9721, 56) -> (123.9721, 51)
  line L688 (128.9721, 56) -> (123.9721, 56)
  line L689 (128.9721, 51) -> (128.9721, 56)
  line L690 (123.9721, 51) -> (128.9721, 51)
  line L691 (107.9721, 51) -> (107.9721, 56)
  line L692 (109.9721, 56) -> (109.9721, 51)
  line L693 (109.9721, 51) -> (114.9721, 51)
  line L694 (114.9721, 51) -> (114.9721, 56)
  line L695 (114.9721, 56) -> (109.9721, 56)
  line L696 (102.9721, 51) -> (107.9721, 51)
  line L697 (95.9721, 51) -> (100.9721, 51)
  line L698 (107.9721, 56) -> (102.9721, 56)
  line L699 (102.9721, 56) -> (102.9721, 51)
  line L700 (100.9721, 51) -> (100.9721, 56)
  line L701 (95.9721, 56) -> (95.9721, 51)
  line L702 (100.9721, 56) -> (95.9721, 56)
  line L703 (88.9721, 51) -> (93.9721, 51)
  line L704 (86.9721, 51) -> (86.9721, 56)
  line L705 (88.9721, 56) -> (88.9721, 51)
  line L706 (93.9721, 56) -> (88.9721, 56)
  line L707 (93.9721, 51) -> (93.9721, 56)
  line L708 (81.9721, 51) -> (86.9721, 51)
  line L709 (81.9721, 56) -> (81.9721, 51)
  line L710 (86.9721, 56) -> (81.9721, 56)
  line L711 (79.9721, 51) -> (79.9721, 56)
  line L712 (74.9721, 51) -> (79.9721, 51)
  line L713 (79.9721, 56) -> (74.9721, 56)
  line L714 (67.9721, 51) -> (72.9721, 51)
  line L715 (67.9721, 56) -> (67.9721, 51)
  line L716 (72.9721, 56) -> (67.9721, 56)
  line L717 (72.9721, 51) -> (72.9721, 56)
  line L718 (74.9721, 56) -> (74.9721, 51)
  line L719 (151.9721, 51) -> (156.9721, 51)
  line L720 (156.9721, 56) -> (151.9721, 56)
  line L721 (156.9721, 51) -> (156.9721, 56)
  line L722 (142.9721, 63) -> (137.9721, 63)
  line L723 (142.9721, 58) -> (142.9721, 63)
  line L724 (137.9721, 58) -> (142.9721, 58)
  line L725 (144.9721, 58) -> (149.9721, 58)
  line L726 (144.9721, 63) -> (144.9721, 58)
  line L727 (149.9721, 58) -> (149.9721, 63)
  line L728 (149.9721, 63) -> (144.9721, 63)
  line L729 (137.9721, 63) -> (137.9721, 58)
  line L730 (130.9721, 58) -> (135.9721, 58)
  line L731 (135.9721, 58) -> (135.9721, 63)
  line L732 (135.9721, 63) -> (130.9721, 63)
  line L733 (130.9721, 63) -> (130.9721, 58)
  line L734 (128.9721, 58) -> (128.9721, 63)
  line L735 (123.9721, 58) -> (128.9721, 58)
  line L736 (128.9721, 63) -> (123.9721, 63)
  line L737 (123.9721, 63) -> (123.9721, 58)
  line L738 (121.9721, 58) -> (121.9721, 63)
  line L739 (109.9721, 58) -> (114.9721, 58)
  line L740 (116.9721, 58) -> (121.9721, 58)
  line L741 (116.9721, 63) -> (116.9721, 58)
  line L742 (114.9721, 58) -> (114.9721, 63)
  line L743 (121.9721, 63) -> (116.9721, 63)
  line L744 (114.9721, 63) -> (109.9721, 63)
  line L745 (102.9721, 58) -> (107.9721, 58)
  line L746 (107.9721, 63) -> (102.9721, 63)
  line L747 (107.9721, 58) -> (107.9721, 63)
  line L748 (109.9721, 63) -> (109.9721, 58)
  line L749 (95.9721, 58) -> (100.9721, 58)
  line L750 (95.9721, 63) -> (95.9721, 58)
  line L751 (100.9721, 58) -> (100.9721, 63)
  line L752 (100.9721, 63) -> (95.9721, 63)
  line L753 (102.9721, 63) -> (102.9721, 58)
  line L754 (88.9721, 58) -> (93.9721, 58)
  line L755 (93.9721, 58) -> (93.9721, 63)
  line L756 (93.9721, 63) -> (88.9721, 63)
  line L757 (81.9721, 58) -> (86.9721, 58)
  line L758 (88.9721, 63) -> (88.9721, 58)
  line L759 (86.9721, 58) -> (86.9721, 63)
  line L760 (81.9721, 63) -> (81.9721, 58)
  line L761 (86.9721, 63) -> (81.9721, 63)
  line L762 (74.9721, 63) -> (74.9721, 58)
  line L763 (67.9721, 58) -> (72.9721, 58)
  line L764 (72.9721, 58) -> (72.9721, 63)
  line L765 (67.9721, 63) -> (67.9721, 58)
  line L766 (72.9721, 63) -> (67.9721, 63)
  line L767 (60.9721, 58) -> (65.9721, 58)
  line L768 (65.9721, 58) -> (65.9721, 63)
  line L769 (65.9721, 63) -> (60.9721, 63)
  line L770 (53.9721, 58) -> (58.9721, 58)
  line L771 (60.9721, 63) -> (60.9721, 58)
  line L772 (58.9721, 58) -> (58.9721, 63)
  line L773 (53.9721, 63) -> (53.9721, 58)
  line L774 (58.9721, 63) -> (53.9721, 63)
  line L775 (39.9721, 58) -> (44.9721, 58)
  line L776 (46.9721, 58) -> (51.9721, 58)
  line L777 (39.9721, 63) -> (39.9721, 58)
  line L778 (44.9721, 63) -> (39.9721, 63)
  line L779 (44.9721, 58) -> (44.9721, 63)
  line L780 (46.9721, 63) -> (46.9721, 58)
  line L781 (51.9721, 63) -> (46.9721, 63)
  line L782 (51.9721, 58) -> (51.9721, 63)
  line L783 (37.9721, 58) -> (37.9721, 63)
  line L784 (37.9721, 63) -> (32.9721, 63)
  line L785 (32.9721, 58) -> (37.9721, 58)
  line L786 (32.9721, 63) -> (32.9721, 58)
  line L787 (79.9721, 58) -> (79.9721, 63)
  line L788 (79.9721, 63) -> (74.9721, 63)
  line L789 (74.9721, 58) -> (79.9721, 58)
  line L790 (121.9721, -2) -> (116.9721, -2)
  line L791 (116.9721, -7) -> (121.9721, -7)
  line L792 (121.9721, -7) -> (121.9721, -2)
  line L793 (114.9721, -2) -> (109.9721, -2)
  line L794 (116.9721, -2) -> (116.9721, -7)
  line L795 (114.9721, -7) -> (114.9721, -2)
  line L796 (109.9721, -7) -> (114.9721, -7)
  line L797 (109.9721, -2) -> (109.9721, -7)
  line L798 (123.9721, -7) -> (128.9721, -7)
  line L799 (128.9721, -7) -> (128.9721, -2)
  line L800 (128.9721, -2) -> (123.9721, -2)
  line L801 (123.9721, -2) -> (123.9721, -7)
  line L802 (142.9721, -7) -> (142.9721, -2)
  line L803 (142.9721, -2) -> (137.9721, -2)
  line L804 (137.9721, -7) -> (142.9721, -7)
  line L805 (137.9721, -2) -> (137.9721, -7)
  line L806 (135.9721, -7) -> (135.9721, -2)
  line L807 (135.9721, -2) -> (130.9721, -2)
  line L808 (130.9721, -2) -> (130.9721, -7)
  line L809 (130.9721, -7) -> (135.9721, -7)
  line L810 (170.9721, -7) -> (170.9721, -2)
  line L811 (170.9721, -2) -> (165.9721, -2)
  line L812 (172.9721, -2) -> (172.9721, -7)
  line L813 (177.9721, -7) -> (177.9721, -2)
  line L814 (177.9721, -2) -> (172.9721, -2)
  line L815 (172.9721, -7) -> (177.9721, -7)
  line L816 (165.9721, -7) -> (170.9721, -7)
  line L817 (151.9721, -7) -> (156.9721, -7)
  line L818 (156.9721, -7) -> (156.9721, -2)
  line L819 (156.9721, -2) -> (151.9721, -2)
  line L820 (151.9721, -2) -> (151.9721, -7)
  line L821 (163.9721, -7) -> (163.9721, -2)
  line L822 (158.9721, -7) -> (163.9721, -7)
  line L823 (163.9721, -2) -> (158.9721, -2)
  line L824 (158.9721, -2) -> (158.9721, -7)
  line L825 (165.9721, -2) -> (165.9721, -7)
  line L826 (95.9721, -7) -> (100.9721, -7)
  line L827 (100.9721, -7) -> (100.9721, -2)
  line L828 (100.9721, -2) -> (95.9721, -2)
  line L829 (95.9721, -2) -> (95.9721, -7)
  line L830 (102.9721, -7) -> (107.9721, -7)
  line L831 (107.9721, -7) -> (107.9721, -2)
  line L832 (107.9721, -2) -> (102.9721, -2)
  line L833 (102.9721, -2) -> (102.9721, -7)
  line L834 (144.9721, -2) -> (144.9721, -7)
  line L835 (144.9721, -7) -> (149.9721, -7)
  line L836 (149.9721, -7) -> (149.9721, -2)
  line L837 (149.9721, -2) -> (144.9721, -2)
  line L838 (144.9721, -9) -> (144.9721, -14)
  line L839 (149.9721, -9) -> (144.9721, -9)
  line L840 (144.9721, -14) -> (149.9721, -14)
  line L841 (149.9721, -14) -> (149.9721, -9)
  line L842 (121.9721, -9) -> (116.9721, -9)
  line L843 (116.9721, -14) -> (121.9721, -14)
  line L844 (121.9721, -14) -> (121.9721, -9)
  line L845 (123.9721, -14) -> (128.9721, -14)
  line L846 (128.9721, -14) -> (128.9721, -9)
  line L847 (128.9721, -9) -> (123.9721, -9)
  line L848 (123.9721, -9) -> (123.9721, -14)
  line L849 (142.9721, -14) -> (142.9721, -9)
  line L850 (142.9721, -9) -> (137.9721, -9)
  line L851 (137.9721, -14) -> (142.9721, -14)
  line L852 (137.9721, -9) -> (137.9721, -14)
  line L853 (135.9721, -14) -> (135.9721, -9)
  line L854 (130.9721, -9) -> (130.9721, -14)
  line L855 (130.9721, -14) -> (135.9721, -14)
  line L856 (135.9721, -9) -> (130.9721, -9)
  line L857 (100.9721, -9) -> (95.9721, -9)
  line L858 (107.9721, -9) -> (102.9721, -9)
  line L859 (114.9721, -9) -> (109.9721, -9)
  line L860 (95.9721, -9) -> (95.9721, -14)
  line L861 (95.9721, -14) -> (100.9721, -14)
  line L862 (100.9721, -14) -> (100.9721, -9)
  line L863 (102.9721, -9) -> (102.9721, -14)
  line L864 (107.9721, -14) -> (107.9721, -9)
  line L865 (109.9721, -9) -> (109.9721, -14)
  line L866 (114.9721, -14) -> (114.9721, -9)
  line L867 (109.9721, -14) -> (114.9721, -14)
  line L868 (116.9721, -9) -> (116.9721, -14)
  line L869 (102.9721, -14) -> (107.9721, -14)
  line L870 (144.9721, -16) -> (144.9721, -21)
  line L871 (149.9721, -16) -> (144.9721, -16)
  line L872 (144.9721, -21) -> (149.9721, -21)
  line L873 (149.9721, -21) -> (149.9721, -16)
  line L874 (121.9721, -16) -> (116.9721, -16)
  line L875 (116.9721, -21) -> (121.9721, -21)
  line L876 (121.9721, -21) -> (121.9721, -16)
  line L877 (123.9721, -21) -> (128.9721, -21)
  line L878 (128.9721, -21) -> (128.9721, -16)
  line L879 (128.9721, -16) -> (123.9721, -16)
  line L880 (123.9721, -16) -> (123.9721, -21)
  line L881 (142.9721, -21) -> (142.9721, -16)
  line L882 (142.9721, -16) -> (137.9721, -16)
  line L883 (137.9721, -21) -> (142.9721, -21)
  line L884 (137.9721, -16) -> (137.9721, -21)
  line L885 (135.9721, -21) -> (135.9721, -16)
  line L886 (130.9721, -16) -> (130.9721, -21)
  line L887 (130.9721, -21) -> (135.9721, -21)
  line L888 (135.9721, -16) -> (130.9721, -16)
  line L889 (100.9721, -16) -> (95.9721, -16)
  line L890 (107.9721, -16) -> (102.9721, -16)
  line L891 (114.9721, -16) -> (109.9721, -16)
  line L892 (95.9721, -16) -> (95.9721, -21)
  line L893 (95.9721, -21) -> (100.9721, -21)
  line L894 (100.9721, -21) -> (100.9721, -16)
  line L895 (102.9721, -16) -> (102.9721, -21)
  line L896 (107.9721, -21) -> (107.9721, -16)
  line L897 (109.9721, -16) -> (109.9721, -21)
  line L898 (114.9721, -21) -> (114.9721, -16)
  line L899 (109.9721, -21) -> (114.9721, -21)
  line L900 (116.9721, -16) -> (116.9721, -21)
  line L901 (102.9721, -21) -> (107.9721, -21)
  line L902 (144.9721, -23) -> (144.9721, -28)
  line L903 (149.9721, -23) -> (144.9721, -23)
  line L904 (144.9721, -28) -> (149.9721, -28)
  line L905 (149.9721, -28) -> (149.9721, -23)
  line L906 (121.9721, -23) -> (116.9721, -23)
  line L907 (116.9721, -28) -> (121.9721, -28)
  line L908 (121.9721, -28) -> (121.9721, -23)
  line L909 (123.9721, -28) -> (128.9721, -28)
  line L910 (128.9721, -28) -> (128.9721, -23)
  line L911 (128.9721, -23) -> (123.9721, -23)
  line L912 (123.9721, -23) -> (123.9721, -28)
  line L913 (142.9721, -28) -> (142.9721, -23)
  line L914 (142.9721, -23) -> (137.9721, -23)
  line L915 (137.9721, -28) -> (142.9721, -28)
  line L916 (137.9721, -23) -> (137.9721, -28)
  line L917 (135.9721, -28) -> (135.9721, -23)
  line L918 (130.9721, -23) -> (130.9721, -28)
  line L919 (130.9721, -28) -> (135.9721, -28)
  line L920 (135.9721, -23) -> (130.9721, -23)
  line L921 (100.9721, -23) -> (95.9721, -23)
  line L922 (107.9721, -23) -> (102.9721, -23)
  line L923 (114.9721, -23) -> (109.9721, -23)
  line L924 (95.9721, -23) -> (95.9721, -28)
  line L925 (95.9721, -28) -> (100.9721, -28)
  line L926 (100.9721, -28) -> (100.9721, -23)
  line L927 (102.9721, -23) -> (102.9721, -28)
  line L928 (107.9721, -28) -> (107.9721, -23)
  line L929 (109.9721, -23) -> (109.9721, -28)
  line L930 (114.9721, -28) -> (114.9721, -23)
  line L931 (109.9721, -28) -> (114.9721, -28)
  line L932 (116.9721, -23) -> (116.9721, -28)
  line L933 (102.9721, -28) -> (107.9721, -28)
  line L934 (144.9721, -30) -> (144.9721, -35)
  line L935 (149.9721, -30) -> (144.9721, -30)
  line L936 (144.9721, -35) -> (149.9721, -35)
  line L937 (149.9721, -35) -> (149.9721, -30)
  line L938 (121.9721, -30) -> (116.9721, -30)
  line L939 (116.9721, -35) -> (121.9721, -35)
  line L940 (121.9721, -35) -> (121.9721, -30)
  line L941 (123.9721, -35) -> (128.9721, -35)
  line L942 (128.9721, -35) -> (128.9721, -30)
  line L943 (128.9721, -30) -> (123.9721, -30)
  line L944 (123.9721, -30) -> (123.9721, -35)
  line L945 (142.9721, -35) -> (142.9721, -30)
  line L946 (142.9721, -30) -> (137.9721, -30)
  line L947 (137.9721, -35) -> (142.9721, -35)
  line L948 (137.9721, -30) -> (137.9721, -35)
  line L949 (135.9721, -35) -> (135.9721, -30)
  line L950 (130.9721, -30) -> (130.9721, -35)
  line L951 (130.9721, -35) -> (135.9721, -35)
  line L952 (135.9721, -30) -> (130.9721, -30)
  line L953 (100.9721, -30) -> (95.9721, -30)
  line L954 (107.9721, -30) -> (102.9721, -30)
  line L955 (114.9721, -30) -> (109.9721, -30)
  line L956 (95.9721, -30) -> (95.9721, -35)
  line L957 (95.9721, -35) -> (100.9721, -35)
  line L958 (100.9721, -35) -> (100.9721, -30)
  line L959 (102.9721, -30) -> (102.9721, -35)
  line L960 (107.9721, -35) -> (107.9721, -30)
  line L961 (109.9721, -30) -> (109.9721, -35)
  line L962 (114.9721, -35) -> (114.9721, -30)
  line L963 (109.9721, -35) -> (114.9721, -35)
  line L964 (116.9721, -30) -> (116.9721, -35)
  line L965 (102.9721, -35) -> (107.9721, -35)
  line L966 (144.9721, -37) -> (144.9721, -42)
  line L967 (149.9721, -37) -> (144.9721, -37)
  line L968 (144.9721, -42) -> (149.9721, -42)
  line L969 (149.9721, -42) -> (149.9721, -37)
  line L970 (121.9721, -37) -> (116.9721, -37)
  line L971 (116.9721, -42) -> (121.9721, -42)
  line L972 (121.9721, -42) -> (121.9721, -37)
  line L973 (123.9721, -42) -> (128.9721, -42)
  line L974 (128.9721, -42) -> (128.9721, -37)
  line L975 (128.9721, -37) -> (123.9721, -37)
  line L976 (123.9721, -37) -> (123.9721, -42)
  line L977 (142.9721, -42) -> (142.9721, -37)
  line L978 (142.9721, -37) -> (137.9721, -37)
  line L979 (137.9721, -42) -> (142.9721, -42)
  line L980 (137.9721, -37) -> (137.9721, -42)
  line L981 (135.9721, -42) -> (135.9721, -37)
  line L982 (130.9721, -37) -> (130.9721, -42)
  line L983 (130.9721, -42) -> (135.9721, -42)
  line L984 (135.9721, -37) -> (130.9721, -37)
  line L985 (100.9721, -37) -> (95.9721, -37)
  line L986 (107.9721, -37) -> (102.9721, -37)
  line L987 (114.9721, -37) -> (109.9721, -37)
  line L988 (95.9721, -37) -> (95.9721, -42)
  line L989 (95.9721, -42) -> (100.9721, -42)
  line L990 (100.9721, -42) -> (100.9721, -37)
  line L991 (102.9721, -37) -> (102.9721, -42)
  line L992 (107.9721, -42) -> (107.9721, -37)
  line L993 (109.9721, -37) -> (109.9721, -42)
  line L994 (114.9721, -42) -> (114.9721, -37)
  line L995 (109.9721, -42) -> (114.9721, -42)
  line L996 (116.9721, -37) -> (116.9721, -42)
  line L997 (102.9721, -42) -> (107.9721, -42)
  line L998 (144.9721, -44) -> (144.9721, -49)
  line L999 (149.9721, -44) -> (144.9721, -44)
  line L1000 (144.9721, -49) -> (149.9721, -49)
  line L1001 (149.9721, -49) -> (149.9721, -44)
  line L1002 (121.9721, -44) -> (116.9721, -44)
  line L1003 (116.9721, -49) -> (121.9721, -49)
  line L1004 (121.9721, -49) -> (121.9721, -44)
  line L1005 (123.9721, -49) -> (128.9721, -49)
  line L1006 (128.9721, -49) -> (128.9721, -44)
  line L1007 (128.9721, -44) -> (123.9721, -44)
  line L1008 (123.9721, -44) -> (123.9721, -49)
  line L1009 (142.9721, -49) -> (142.9721, -44)
  line L1010 (142.9721, -44) -> (137.9721, -44)
  line L1011 (137.9721, -49) -> (142.9721, -49)
  line L1012 (137.9721, -44) -> (137.9721, -49)
  line L1013 (135.9721, -49) -> (135.9721, -44)
  line L1014 (130.9721, -44) -> (130.9721, -49)
  line L1015 (130.9721, -49) -> (135.9721, -49)
  line L1016 (135.9721, -44) -> (130.9721, -44)
  line L1017 (100.9721, -44) -> (95.9721, -44)
  line L1018 (107.9721, -44) -> (102.9721, -44)
  line L1019 (114.9721, -44) -> (109.9721, -44)
  line L1020 (95.9721, -44) -> (95.9721, -49)
  line L1021 (95.9721, -49) -> (100.9721, -49)
  line L1022 (100.9721, -49) -> (100.9721, -44)
  line L1023 (102.9721, -44) -> (102.9721, -49)
  line L1024 (107.9721, -49) -> (107.9721, -44)
  line L1025 (109.9721, -44) -> (109.9721, -49)
  line L1026 (114.9721, -49) -> (114.9721, -44)
  line L1027 (109.9721, -49) -> (114.9721, -49)
  line L1028 (116.9721, -44) -> (116.9721, -49)
  line L1029 (102.9721, -49) -> (107.9721, -49)
  line L1030 (144.9721, -51) -> (144.9721, -56)
  line L1031 (149.9721, -51) -> (144.9721, -51)
  line L1032 (144.9721, -56) -> (149.9721, -56)
  line L1033 (149.9721, -56) -> (149.9721, -51)
  line L1034 (121.9721, -51) -> (116.9721, -51)
  line L1035 (116.9721, -56) -> (121.9721, -56)
  line L1036 (121.9721, -56) -> (121.9721, -51)
  line L1037 (123.9721, -56) -> (128.9721, -56)
  line L1038 (128.9721, -56) -> (128.9721, -51)
  line L1039 (128.9721, -51) -> (123.9721, -51)
  line L1040 (123.9721, -51) -> (123.9721, -56)
  line L1041 (142.9721, -56) -> (142.9721, -51)
  line L1042 (142.9721, -51) -> (137.9721, -51)
  line L1043 (137.9721, -56) -> (142.9721, -56)
  line L1044 (137.9721, -51) -> (137.9721, -56)
  line L1045 (135.9721, -56) -> (135.9721, -51)
  line L1046 (130.9721, -51) -> (130.9721, -56)
  line L1047 (130.9721, -56) -> (135.9721, -56)
  line L1048 (135.9721, -51) -> (130.9721, -51)
  line L1049 (100.9721, -51) -> (95.9721, -51)
  line L1050 (107.9721, -51) -> (102.9721, -51)
  line L1051 (114.9721, -51) -> (109.9721, -51)
  line L1052 (95.9721, -51) -> (95.9721, -56)
  line L1053 (95.9721, -56) -> (100.9721, -56)
  line L1054 (100.9721, -56) -> (100.9721, -51)
  line L1055 (102.9721, -51) -> (102.9721, -56)
  line L1056 (107.9721, -56) -> (107.9721, -51)
  line L1057 (109.9721, -51) -> (109.9721, -56)
  line L1058 (114.9721, -56) -> (114.9721, -51)
  line L1059 (109.9721, -56) -> (114.9721, -56)
  line L1060 (116.9721, -51) -> (116.9721, -56)
  line L1061 (102.9721, -56) -> (107.9721, -56)
  line L1062 (144.9721, -58) -> (144.9721, -63)
  line L1063 (149.9721, -58) -> (144.9721, -58)
  line L1064 (144.9721, -63) -> (149.9721, -63)
  line L1065 (149.9721, -63) -> (149.9721, -58)
  line L1066 (121.9721, -58) -> (116.9721, -58)
  line L1067 (116.9721, -63) -> (121.9721, -63)
  line L1068 (121.9721, -63) -> (121.9721, -58)
  line L1069 (123.9721, -63) -> (128.9721, -63)
  line L1070 (128.9721, -63) -> (128.9721, -58)
  line L1071 (128.9721, -58) -> (123.9721, -58)
  line L1072 (123.9721, -58) -> (123.9721, -63)
  line L1073 (142.9721, -63) -> (142.9721, -58)
  line L1074 (142.9721, -58) -> (137.9721, -58)
  line L1075 (137.9721, -63) -> (142.9721, -63)
  line L1076 (137.9721, -58) -> (137.9721, -63)
  line L1077 (135.9721, -63) -> (135.9721, -58)
  line L1078 (130.9721, -58) -> (130.9721, -63)
  line L1079 (130.9721, -63) -> (135.9721, -63)
  line L1080 (135.9721, -58) -> (130.9721, -58)
  line L1081 (100.9721, -58) -> (95.9721, -58)
  line L1082 (107.9721, -58) -> (102.9721, -58)
  line L1083 (114.9721, -58) -> (109.9721, -58)
  line L1084 (95.9721, -58) -> (95.9721, -63)
  line L1085 (95.9721, -63) -> (100.9721, -63)
  line L1086 (100.9721, -63) -> (100.9721, -58)
  line L1087 (102.9721, -58) -> (102.9721, -63)
  line L1088 (107.9721, -63) -> (107.9721, -58)
  line L1089 (109.9721, -58) -> (109.9721, -63)
  line L1090 (114.9721, -63) -> (114.9721, -58)
  line L1091 (109.9721, -63) -> (114.9721, -63)
  line L1092 (116.9721, -58) -> (116.9721, -63)
  line L1093 (102.9721, -63) -> (107.9721, -63)
  line L1094 (100.9721, -65) -> (95.9721, -65)
  line L1095 (95.9721, -70) -> (100.9721, -70)